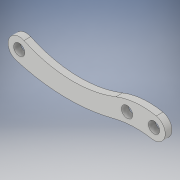
# Autodesk Inventor part: panto_linkagedi
Saved by Autodesk Inventor 2017 (Build 210142000, 142)
## iProperties
Created: 2016-08-20
Part Number: panto_linkagedi
Material: Generic
Document SubType Name: Modeling
Designer: Nic
Density: 1 g/cm^3
Appearance: Default
Author: Nic
Autodesk Inventor part; units mm, degrees
ref_plane "YZ Plane" through (0, 0, 0) normal (1, 0, 0) x (0, 1, 0)
ref_plane "XZ Plane" through (0, 0, 0) normal (0, 1, 0) x (-1, 0, 0)
ref_plane "XY Plane" through (0, 0, 0) normal (0, 0, 1) x (1, 0, 0)
sketch "Sketch1" plane through (0, 0, 0) normal (0, 0, 1) x (1, 0, 0)
  circle A0 centre (0, 0) radius 1.25
  line L0 (0, 0) -> (24, 0) construction
  circle A1 centre (24, 0) radius 1.25
  arc A2 (1.0526, 2.2676) -> (-0.7212, -2.3937) centre (0, 0) ccw
  circle A3 centre (30, 0) radius 1.25
  line L1 (17.5, 0) -> (17.5, 10) construction
  arc A4 (1.0526, 2.2676) -> (21.5093, 1.6519) centre (12, 25.8505) ccw
  arc A5 (30.4887, 2.4518) -> (21.5093, 1.6519) centre (27.3611, -13.2396) ccw
  arc A6 (29.5556, -2.4602) -> (30.4887, 2.4518) centre (30, 0) ccw
  arc A7 (-0.7212, -2.3937) -> (20.9392, -2.7925) centre (10.8177, 35.9058) ccw
  arc A8 (29.5556, -2.4602) -> (20.9392, -2.7925) centre (26, -22.1416) ccw
  dimension "d0" = 2.5
  dimension "d1" = 24
  dimension "d8" = 5
  dimension "d16" = 30
  dimension "d17" = 10
  dimension "d18" = 17.5
  dimension "d20" = 5
  dimension "d21" = 26
  dimension "d22" = 40
  dimension "d23" = 16
  dimension "d24" = 20
  dimension "d25" = 12
  dimension "d26" = 26
  constraints: 15 point on circle, 9 centre point, 6 tangent, 4 coincident, 4 end point, 2 equal radius, 1 horizontal, 1 horizontal alignment, 1 point on line, 1 vertical
  measures "d0" diameter of A0
  measures "d1" distance of L0.start L0.end
  measures "d8" diameter of A2
  measures "d16" distance of point (0, 0) A3.centre
  measures "d17" distance of L1.start L1.end
  measures "d18" distance from line of point (0, 0) L1
  measures "d20" diameter of A6
  measures "d21" radius of A4
  measures "d22" radius of A7
  measures "d23" radius of A5
  measures "d24" radius of A8
  measures "d25" horizontal distance of point (0, 0) A4.centre
  measures "d26" horizontal distance of point (0, 0) A8.centre
extrude "Extrusion1" add sketch "Sketch1" along normal blind 1.5
body "Solid1"
